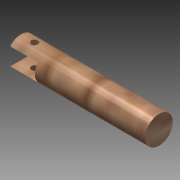
# Autodesk Inventor part: 曲柄杆
Saved by Autodesk Inventor 2013 (Build 170138000, 138)
## iProperties
Created: 2012-10-03
Part Number: 曲柄杆
Material: 木材(桦木)
Document SubType Name: Modeling
Designer: Zhensheng
Density: 7.85 g/cm^3
Author: Zhensheng
Autodesk Inventor part; units mm, degrees
ref_plane "YZ Plane" through (0, 0, 0) normal (1, 0, 0) x (0, 1, 0)
ref_plane "XZ Plane" through (0, 0, 0) normal (0, 1, 0) x (-1, 0, 0)
ref_plane "XY Plane" through (0, 0, 0) normal (0, 0, 1) x (1, 0, 0)
sketch "草图1" plane through (0, 0, 0) normal (1, 0, 0) x (0, 1, 0)
  circle A0 centre (0, 0) radius 2
  dimension "孔径" = 4
  constraints: 1 centre point, 1 coincident
  measures "孔径" diameter of A0
extrude "拉伸1" add sketch "草图1" along normal blind 20
sketch "草图2" plane through (0, 0, 0) normal (0, 1, 0) x (-1, 0, 0)
  line L0 (-20, 2) -> (-20, -2) projected
  line L1 (0, -2) -> (0, 2) projected
  line L2 (0, 2) -> (-20, 2) projected
  line L3 (-4, 2) -> (-4, -2)
  line L4 (0, 0) -> (-4, 0) construction
  line L5 (0, 1.25) -> (-4, 1.25)
  line L6 (0, -1.25) -> (-4, -1.25)
  dimension "d4" = 4
  dimension "距离" = 2.5
  constraints: 8 end point, 5 point on line, 1 midpoint, 1 other
  measures "d4" distance between parallel lines of L1 L3
  measures "距离" distance between parallel lines of L6 L5
extrude "拉伸2" cut sketch "草图2" along normal through all both and the other way through all contours L6 L3 L5 L1
sketch "草图3" plane through (0, 0, 0) normal (0, 0, 1) x (1, 0, 0)
  line L0 (4, -1.5612) -> (0, -1.5612) projected
  line L1 (4, -1.5612) -> (4, 1.5612) projected
  line L2 (0, 1.5612) -> (4, 1.5612) projected
  line L3 (0, -1.5612) -> (0, 1.5612) projected
  circle A0 centre (2, 0) radius 0.5
  point P0 (0, 0)
  dimension "销孔径" = 1
  constraints: 1 centre point, 1 coincident, 1 other
  measures "销孔径" diameter of A0
extrude "拉伸3" cut sketch "草图3" along normal through all both and the other way through all contours A0
